Autodesk Fusion 360 part; units mm, degrees
(part 2 of 2)
sketch "Sketch8" plane through (0, 0, 4) normal (0, 0, 1) x (-1, 0, 0)
  circle A0 centre (-33.2439, -40.7427) radius 1.6
  circle A1 centre (-15.5775, -40.6826) radius 1.6
  line L0 (-39.5332, 26.8536) -> (-36.9332, 25.3524)
  line L1 (-36.9332, 25.3524) -> (-36.9332, 22.3502)
  line L2 (-36.9332, 22.3502) -> (-39.5332, 20.8491)
  line L3 (-39.5332, 20.8491) -> (-42.1332, 22.3502)
  line L4 (-42.1332, 22.3502) -> (-42.1332, 25.3524)
  line L5 (-42.1332, 25.3524) -> (-39.5332, 26.8536)
  line L6 (-9.3909, 26.6177) -> (-6.7825, 25.1314)
  line L7 (-6.7825, 25.1314) -> (-6.7654, 22.1292)
  line L8 (-6.7654, 22.1292) -> (-9.3568, 20.6133)
  line L9 (-9.3568, 20.6133) -> (-11.9653, 22.0997)
  line L10 (-11.9653, 22.0997) -> (-11.9824, 25.1018)
  line L11 (-11.9824, 25.1018) -> (-9.3909, 26.6177)
  line L12 (-50, 11) -> (-50, -26)
  line L13 (-50, -26) -> (-73.2304, -26)
  line L14 (-73.2304, -26) -> (-73.2304, 11)
  line L15 (-73.2304, 11) -> (-50, 11)
  line L16 (-50, -33) -> (-50, -45.3866)
  line L17 (-50, -45.3866) -> (-73.2304, -45.3866)
  line L18 (-73.2304, -45.3866) -> (-73.2304, -33)
  line L19 (-73.2304, -33) -> (-50, -33)
  line L20 (-1, -45.3866) -> (-1, -25)
  line L21 (-1, -25) -> (19.7696, -25)
  line L22 (19.7696, -25) -> (19.7696, -45.3866)
  line L23 (19.7696, -45.3866) -> (-1, -45.3866)
  line L24 (-1, -18) -> (-1, 11)
  line L25 (-1, 11) -> (19.7696, 11)
  line L26 (19.7696, 11) -> (19.7696, -18)
  line L27 (19.7696, -18) -> (-1, -18)
  line L28 (-1, 18) -> (-1, 30.587)
  line L29 (-1, 30.587) -> (19.7696, 30.587)
  line L30 (19.7696, 30.587) -> (19.7696, 18)
  line L31 (19.7696, 18) -> (-1, 18)
  arc A2 (-79.2313, 37.6134) -> (-80.2313, 36.6134) centre (-79.2313, 36.6134) ccw
  line L32 (-80.2313, 36.6134) -> (-80.2313, -51.3866)
  arc A3 (-80.2313, -51.3866) -> (-79.2313, -52.3866) centre (-79.2313, -51.3866) ccw
  line L33 (-79.2313, -52.3866) -> (25.7696, -52.3866)
  arc A4 (25.7696, -52.3866) -> (26.7696, -51.3866) centre (25.7696, -51.3866) ccw
  line L34 (26.7696, -51.3866) -> (26.7696, 36.6134)
  arc A5 (26.7696, 36.6134) -> (25.7696, 37.6134) centre (25.7696, 36.6134) ccw
  line L35 (25.7696, 37.6134) -> (-79.2313, 37.6134)
  circle A6 centre (-66.7314, 34.1104) radius 1.5
  circle A7 centre (13.2753, 34.1171) radius 1.5
  circle A8 centre (13.2624, -48.8983) radius 1.5
  circle A9 centre (-66.7239, -48.8933) radius 1.5
  line L36 (-50, 18) -> (-73.2304, 18)
  line L37 (-73.2304, 18) -> (-73.2304, 30.587)
  line L38 (-73.2304, 30.587) -> (-50, 30.587)
  line L39 (-50, 30.587) -> (-50, 18)
  line L40 (-35.9985, 22.2168) -> (-35.9985, 25.4858)
  line L41 (-35.9985, 25.4858) -> (-13.2, 25.25)
  line L42 (-13.2, 25.25) -> (-13.2, 21.981)
  line L43 (-13.2, 21.981) -> (-35.9985, 22.2168)
  line L44 (-12.7275, -39.0371) -> (-15.5775, -37.3917)
  line L45 (-15.5775, -37.3917) -> (-18.4275, -39.0371)
  line L46 (-18.4275, -39.0371) -> (-18.4275, -42.328)
  line L47 (-18.4275, -42.328) -> (-15.5775, -43.9735)
  line L48 (-15.5775, -43.9735) -> (-12.7275, -42.328)
  line L49 (-12.7275, -42.328) -> (-12.7275, -39.0371)
  line L50 (-30.4118, -39.0668) -> (-33.2793, -37.452)
  line L51 (-33.2793, -37.452) -> (-36.1114, -39.128)
  line L52 (-36.1114, -39.128) -> (-36.0761, -42.4187)
  line L53 (-36.0761, -42.4187) -> (-33.2086, -44.0334)
  line L54 (-33.2086, -44.0334) -> (-30.3764, -42.3575)
  line L55 (-30.3764, -42.3575) -> (-30.4118, -39.0668)
  point P0 (-15.5775, -40.6826)
  point P1 (-33.2439, -40.7427)
  dimension "d66" = 2.85
  dimension "d67" = 2.85
  constraint coincident P0 A1.centre
  constraint coincident A0.centre P1
  measures "d66" distance of P0 L49
  measures "d67" distance of P1 L55
extrude "Extrude10" cut sketch "Sketch8" against normal blind 2.25 contours L44 L45 L46 L47 L48 L49 | L50 L51 L52 L53 L54 L55 bodies 1
sketch "Sketch9" plane through (0, 0, 0) normal (0, 0, 1) x (1, 0, 0)
extrude "Extrude6" cut sketch "Sketch4" against normal blind 2 contours A8 | A9 | A10 | A11 bodies 1
sketch "Sketch10" plane through (0, 0, -3) normal (0, 0, -1) x (1, 0, 0)
  circle A0 centre (39.5332, 23.8513) radius 1.375
  arc A1 (42.4985, 22.2168) -> (42.18, 25.4858) centre (42.4985, 23.8668) ccw
  line L0 (42.18, 25.4858) -> (35.9985, 25.4858)
  line L1 (35.9985, 25.4858) -> (35.9985, 22.2168)
  line L2 (35.9985, 22.2168) -> (42.4985, 22.2168)
  circle A2 centre (39.5332, 23.8513) radius 1.375
  circle A3 centre (9.3739, 23.6155) radius 1.375
  circle A4 centre (15.5775, -40.6826) radius 1.6
  circle A5 centre (33.2439, -40.7427) radius 1.6
  line L3 (9.3739, 23.6155) -> (3.3739, 23.6155) construction
  line L4 (9.3739, 23.6155) -> (9.3739, 29.6155) construction
  line L5 (9.3739, 29.6155) -> (3.3739, 23.6155) construction
  line L6 (33.2439, -40.7427) -> (33.2439, -46.7427) construction
  line L7 (39.5332, 23.8513) -> (39.5332, 29.8513) construction
  line L8 (39.5332, 23.8513) -> (45.5332, 23.8513) construction
  line L9 (45.5332, 23.8513) -> (39.5332, 29.8513) construction
  line L10 (42.5332, 26.8513) -> (42.5332, -43.8397) construction
  line L11 (6.3739, 26.6155) -> (42.5332, 26.6155)
  line L12 (42.5332, 26.6155) -> (42.5332, -43.8397)
  line L13 (42.5332, -43.8397) -> (6.3739, -43.8397)
  line L14 (6.3739, -43.8397) -> (6.3739, 26.6155)
  line L15 (9.3739, 23.6155) -> (9.3739, 17.6155) construction
  line L16 (9.3739, 23.6155) -> (15.3739, 23.6155) construction
  line L17 (39.5332, 23.8513) -> (33.5332, 23.8513) construction
  line L18 (39.5332, 23.8513) -> (39.5332, 17.8513) construction
  line L19 (30.3135, -37.6553) -> (42.5332, -37.6553) construction
  line L20 (37.3114, 20.8513) -> (37.3114, -37.6553) construction
  line L21 (11.7887, 21.8355) -> (37.3114, 21.8355)
  line L22 (37.3114, 21.8355) -> (37.3114, -37.6553)
  line L23 (37.3114, -37.6553) -> (11.7887, -37.6553)
  line L24 (11.7887, -37.6553) -> (11.7887, 21.8355)
  circle A6 centre (33.2439, -40.7427) radius 3 construction
  circle A7 centre (15.5775, -40.6826) radius 3 construction
  circle A8 centre (39.5332, 23.8513) radius 3 construction
  circle A9 centre (9.3739, 23.6155) radius 3 construction
  line L25 (11.7887, 21.8355) -> (11.7887, 26.6155)
  line L26 (37.3114, 21.8355) -> (37.3114, 26.6155)
  line L27 (11.7887, 21.8355) -> (11.7887, 16.8355) construction
  line L28 (11.7887, 16.8355) -> (37.3114, 16.8526)
  dimension "d70" = 6
  dimension "d71" = 6
  dimension "d72" = 6
  dimension "d73" = 6
  dimension "d74" = 6
  dimension "d75" = 6
  dimension "d76" = 6
  dimension "d77" = 6
  dimension "d78" = 6
  dimension "d82" = 6
  dimension "d83" = 6
  dimension "d84" = 6
  dimension "d85" = 6
  dimension "d86" = 5
  constraint concentric A0 A2
  constraint coincident A3.centre L3.start
  constraint horizontal L3
  constraint perpendicular L3 L4
  constraint coincident A5.centre L6.start
  constraint parallel L4 L6
  constraint coincident A0.centre A2.centre
  constraint perpendicular L0 L7
  constraint perpendicular L7 L8
  constraint midpoint L9 L10.start
  constraint horizontal L11
  constraint vertical L12
  constraint horizontal L13
  constraint vertical L14
  constraint midpoint L5 L11.start
  constraint perpendicular L3 L15
  constraint perpendicular L4 L16
  constraint perpendicular L7 L17
  constraint perpendicular L8 L18
  constraint horizontal L19
  constraint coincident L10 L19.end
  constraint coincident L19 L20.end
  constraint perpendicular L19 L20
  constraint horizontal L21
  constraint vertical L22
  constraint horizontal L23
  constraint vertical L24
  constraint concentric A5 A6
  constraint concentric A4 A7
  constraint concentric A2 A8
  constraint coincident L21.start A9
  constraint coincident L21.end A8
  constraint coincident L11 L25.end
  constraint perpendicular L11 L25
  constraint coincident L11 L26.end
  constraint perpendicular L11 L26
  constraint perpendicular L21 L27
  constraint coincident L20 L28.end
  measures "d70" distance of A3.centre L3.end
  measures "d71" distance of A3.centre L4.end
  measures "d72" distance of A5.centre L6.end
  measures "d73" distance of A0.centre L7.end
  measures "d74" distance of A0.centre L8.end
  measures "d75" distance of A3.centre L15.end
  measures "d76" distance of A3.centre L16.end
  measures "d77" distance of A0.centre L17.end
  measures "d78" distance of A0.centre L18.end
  measures "d82" diameter of A6
  measures "d83" diameter of A7
  measures "d84" diameter of A8
  measures "d85" diameter of A9
  measures "d86" distance of L21.start L27.end
extrude "Extrude11" add sketch "Sketch10" along normal blind 4 separate body contours A1 L0 L2 L12 L26 | A1 L2 L11 L12 L13 L14 L22 L23 L24 L25 L26 | L0 L1 L2 L11 L21 L25 L26 | L0 L1 L2 L26 | A1 L0 L11 L12 L26 makes body 2
extrude "Extrude12" add sketch "Sketch10" along normal blind 4 contours L21 L22 L24 L28 bodies 2
extrude "Extrude13" cut sketch "Sketch10" along normal blind 4 contours L0 L1 L2 L11 L21 L25 L26 | L0 L1 L2 L26 bodies 2
